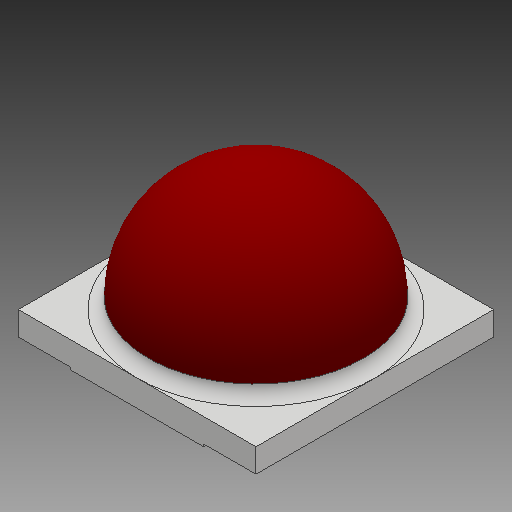
# Autodesk Inventor part: CREE XLamp 1W 5x5
Saved by Autodesk Inventor 2019.1 (Build 231200000, 200)
## iProperties
Part Number: CREE XLamp 1W 5x5
Material: Generisch
Document SubType Name: Modeling
Designer: rYan
Density: 1 g/cm^3
Appearance: Vorgabe
Mass: 0.0414067 g
Surface Area: 0.787969 cm^2
Volume: 0.0414067 cm^3
Author: rYan
Autodesk Inventor part; units mm, degrees
ref_plane "YZ Plane" through (0, 0, 0) normal (1, 0, 0) x (0, 1, 0)
ref_plane "XZ Plane" through (0, 0, 0) normal (0, 1, 0) x (-1, 0, 0)
ref_plane "XY Plane" through (0, 0, 0) normal (0, 0, 1) x (1, 0, 0)
sketch "Skizze1" plane through (0, 0, 0) normal (0, 0, 1) x (1, 0, 0)
  line L0 (-2.5, -2.5) -> (2.5, -2.5)
  line L1 (2.5, -2.5) -> (2.5, 2.5)
  line L2 (2.5, 2.5) -> (-2.5, 2.5)
  line L3 (-2.5, 2.5) -> (-2.5, -2.5)
  line L4 (-2.5, -2.5) -> (2.5, 2.5) construction
  line L5 (2.5, -2.5) -> (-2.5, 2.5) construction
  point P0 (0, 0)
  dimension "d0" = 5
  dimension "d1" = 5
  constraints: 12 end point, 2 midpoint, 2 parallel, 1 horizontal, 1 perpendicular
  measures "d0" distance of L2.end L1.end
  measures "d1" distance of L1.end L0.end
extrude "Extrusion1" add sketch "Skizze1" along normal blind 0.5
sketch "Skizze2" plane through (0, 0, 0) normal (0, 1, 0) x (-1, 0, 0)
  line L0 (2.5, 0) -> (-2.5, 0) projected
  line L1 (-2.5, 0) -> (-2.5, 0.5) projected
  line L2 (2.5, 0.5) -> (-2.5, 0.5) projected
  line L3 (2.5, 0) -> (2.5, 0.5) projected
  line L4 (0, 0.5) -> (0, 3)
  arc A0 (0, 3) -> (-2.26, 0.74) centre (0, 0.74) ccw
  line L5 (-2.5, 0.5) -> (2.5, 0.5) projected
  arc A1 (-2.5, 0.5) -> (-2.26, 0.74) centre (-2.5, 0.74) ccw
  line L6 (0, 0.5) -> (-2.5, 0.5)
  line L7 (0, -0.6936) -> (0, 4.1617) projected
  point P0 (0, 0)
  dimension "d4" = 2.26
  dimension "d5" = 3
  constraints: 4 end point, 4 point on circle, 2 centre point, 2 tangent, 1 midpoint, 1 point on line, 1 vertical
  measures "d4" radius of A0
  measures "d5" distance from line of L4.end L0
revolve "Umdrehung1" add sketch "Skizze2" angle 360 about axis through (0, 0, -10) along (0, 0, 1) contours L2 A1 A0 L4
sketch "Skizze3" plane through (0, 0, 0) normal (0, 0, -1) x (-1, 0, 0)
  line L0 (2.5, -2.5) -> (-2.5, -2.5) projected
  line L1 (2.5, 2.5) -> (2.5, -2.5) projected
  line L2 (-2.5, 2.5) -> (2.5, 2.5) projected
  line L3 (-2.5, -2.5) -> (-2.5, 2.5) projected
  line L4 (2.5, -2.5) -> (-2.5, -2.5) projected
  line L5 (-2.5, 2.5) -> (2.5, 2.5) projected
  line L6 (1.4, -2.5) -> (-1.4, -2.5)
  line L7 (-1.4, -2.5) -> (-1.4, 2.5)
  line L8 (-1.4, 2.5) -> (1.4, 2.5)
  line L9 (1.4, 2.5) -> (1.4, -2.5)
  line L10 (0, -2.5) -> (0, 2.5) construction
  point P0 (0, 0)
  dimension "d7" = 2.8
  constraints: 10 end point, 3 midpoint, 2 parallel, 2 perpendicular, 2 point on line, 1 horizontal, 1 other
  measures "d7" distance between parallel lines of L7 L9
extrude "Extrusion2" add sketch "Skizze3" along normal blind 0.05 contours L0 L7 L2 L9
